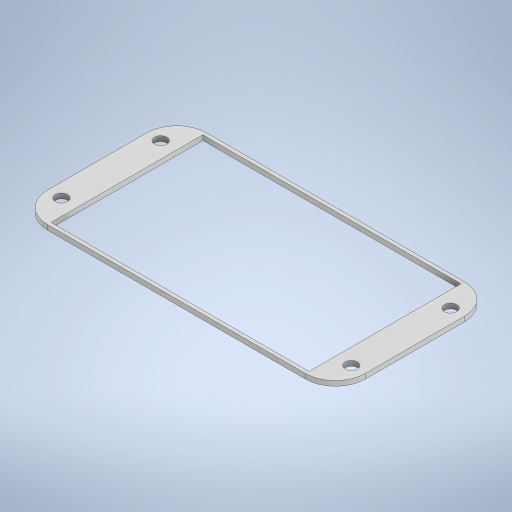
# Autodesk Inventor part: redline
Saved by Autodesk Inventor 2024.3 (Build 283343000, 343)
## iProperties
Created: 2025-08-07
Part Number: redline
Material: Ogólny
Document SubType Name: Modeling
Designer: User
Density: 1 g/cm^3
Appearance: Domyślna
Author: User
Autodesk Inventor part; units mm, degrees
ref_plane "YZ Plane" through (0, 0, 0) normal (1, 0, 0) x (0, 1, 0)
ref_plane "XZ Plane" through (0, 0, 0) normal (0, 1, 0) x (-1, 0, 0)
ref_plane "XY Plane" through (0, 0, 0) normal (0, 0, 1) x (1, 0, 0)
sketch "Szkic1" plane through (0, 0, 0) normal (0, 1, 0) x (-1, 0, 0)
  line L0 (-21.186, -15.0745) -> (-26.186, -15.0745)
  line L1 (-26.186, -15.0745) -> (-26.186, 16.9255)
  line L2 (-26.186, 16.9255) -> (-21.186, 16.9255)
  line L3 (-21.186, 16.9255) -> (-21.186, -15.0745)
  circle A0 centre (-23.386, -9.0745) radius 1.25
  line L4 (-21.186, 0.9255) -> (32.814, 0.9255)
  line L5 (32.814, 16.9255) -> (32.814, -15.0745)
  line L6 (5.814, 0.9255) -> (5.814, -15.0745)
  line L7 (32.814, 16.9255) -> (32.814, -15.0745)
  line L8 (37.814, 16.9255) -> (32.814, 16.9255)
  line L9 (37.814, -15.0745) -> (37.814, 16.9255)
  line L10 (32.814, -15.0745) -> (37.814, -15.0745)
  line L11 (-21.186, 0.9255) -> (-26.186, 0.9255)
  line L12 (-23.386, 0.9255) -> (-23.386, -9.0745)
  line L13 (-23.386, 0.9255) -> (-13.386, 0.9255) construction
  circle A1 centre (-23.386, 10.9255) radius 1.25
  circle A2 centre (35.014, 10.9255) radius 1.25
  circle A3 centre (35.014, -9.0745) radius 1.25
  line L14 (32.814, 16.9255) -> (-21.186, 16.9255)
  line L15 (-21.186, 16.9255) -> (-21.186, -15.0745)
  line L16 (-21.186, -15.0745) -> (32.814, -15.0745)
  line L17 (32.814, -15.0745) -> (32.814, 16.9255)
  line L18 (32.814, 16.9255) -> (-21.186, -15.0745) construction
  line L19 (-21.186, 16.9255) -> (32.814, -15.0745) construction
  line L20 (32.414, -14.3745) -> (-20.186, -14.3745)
  line L21 (31.814, 16.2255) -> (-20.186, 16.2255)
  line L22 (-20.186, 16.2255) -> (-20.186, -14.3745)
  line L23 (-20.186, -14.3745) -> (31.814, -14.3745)
  line L24 (31.814, -14.3745) -> (31.814, 16.2255)
  line L25 (31.814, 16.2255) -> (-20.186, -14.3745) construction
  line L26 (-20.186, 16.2255) -> (31.814, -14.3745) construction
  dimension "d12" = 32
  dimension "d13" = 2.5
  dimension "d14" = 5
  dimension "d15" = 2.2
  dimension "d16" = 10
  dimension "d17" = 90
  constraints: 54 end point, 8 midpoint, 6 parallel, 5 horizontal, 5 symmetric about line, 4 centre point, 4 perpendicular, 2 vertical, 3 other
  measures "d12" distance of L0.end L1.end
  measures "d13" diameter of A0
  measures "d14" distance between parallel lines of L1 L3
  measures "d15" distance from line of L3 A0.centre
  measures "d16" distance of L12.start L12.end
  measures "d17" angle of L12 L13
extrude "Wyciągnięcie proste1" add sketch "Szkic1" along normal blind 1 contours L0 L1 L11 L3 | L3 L4 L22 L20 L6 L16 | L11 L1 L2 L3 | L3 L14 L5 L4 L24 L21 L22 | L6 L20 L24 L4 L5 L16 | L5 L8 L9 L10
fillet "Zaokrąglenie1" radius 6 4 edges at (-37.814, 0.5, 16.9255) (-37.814, 0.5, -15.0745) (26.186, 0.5, -15.0745) (26.186, 0.5, 16.9255)
